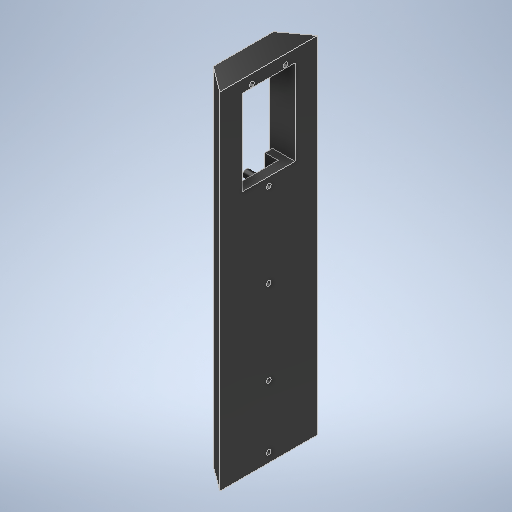
# Autodesk Inventor part: Fullenss sensor v3.1 holder
Saved by Autodesk Inventor 2025 (Build 290162000, 162)
## iProperties
Created: 2025-12-14
Part Number: Fullenss sensor v3.1 holder
Material: Generic
Document SubType Name: Modeling
Designer: kingc
Density: 1 g/cm^3
Appearance: Glossy - Black
Author: kingc
Autodesk Inventor part; units mm, degrees
ref_plane "YZ Plane" through (0, 0, 0) normal (1, 0, 0) x (0, 1, 0)
ref_plane "XZ Plane" through (0, 0, 0) normal (0, 1, 0) x (-1, 0, 0)
ref_plane "XY Plane" through (0, 0, 0) normal (0, 0, 1) x (1, 0, 0)
sketch "Sketch1" plane through (0, 0, 0) normal (1, 0, 0) x (0, 1, 0)
  line L0 (0, 0) -> (228.6, 0)
  line L1 (228.6, 0) -> (228.6, -35.56)
  line L2 (228.6, -35.56) -> (0, -35.56)
  line L3 (0, -35.56) -> (0, 0)
  line L4 (228.6, 0) -> (222.758, 0)
  line L5 (222.758, 0) -> (222.758, -35.56)
  line L6 (222.758, -35.56) -> (228.6, -35.56)
  line L7 (228.6, -35.56) -> (228.6, 0)
  circle A0 centre (224.79, -6.35) radius 1.5875
  circle A1 centre (224.79, -29.21) radius 1.5875
  line L8 (222.758, 0) -> (0, 0)
  line L9 (165.1, -5.08) -> (6.35, -5.08)
  line L10 (6.35, -5.08) -> (6.35, -30.48)
  line L11 (6.35, -30.48) -> (165.1, -30.48)
  line L12 (222.758, -33.02) -> (222.758, -2.54)
  line L13 (165.1, 0) -> (165.1, -35.56)
  line L14 (231.14, 2.54) -> (-2.54, 2.54)
  line L15 (-2.54, 2.54) -> (-2.54, -38.1)
  line L16 (-2.54, -38.1) -> (231.14, -38.1)
  line L17 (231.14, -38.1) -> (231.14, 2.54)
  point P0 (110.998, 0)
  point P1 (228.6, -17.78)
  dimension "d0" = 228.6
  dimension "d1" = 35.56
  dimension "d2" = 5.842
  dimension "d3" = 3.175
  dimension "d4" = 3.175
  dimension "d5" = 3.81
  dimension "d6" = 6.35
  dimension "d7" = 3.81
  dimension "d8" = 6.35
  dimension "d14" = 5.08
  dimension "d15" = 5.08
  dimension "d16" = 6.35
  dimension "d17" = 0
  dimension "d18" = 63.5
  dimension "d19" = 2.54
  dimension "d20" = 2.54
  dimension "d21" = 2.54
  dimension "d22" = 2.54
  constraints: 36 end point, 8 parallel, 7 point on line, 5 horizontal, 5 perpendicular, 2 centre point, 1 midpoint
  measures "d0" distance of L1.end L2.end
  measures "d1" distance of L0.end L1.end
  measures "d2" distance of L6.end L5.end
  measures "d3" diameter of A0
  measures "d4" diameter of A1
  measures "d5" distance from line of L1 A0.centre
  measures "d6" distance from line of L0 A0.centre
  measures "d7" distance from line of L1 A1.centre
  measures "d8" distance from line of L2 A1.centre
  measures "d14" distance between parallel lines of L0 L9
  measures "d15" distance between parallel lines of L2 L11
  measures "d16" distance between parallel lines of L3 L10
  measures "d17" distance between parallel lines of L5 L12
  measures "d18" distance from line of point (228.6, -17.78) L13
  measures "d19" distance between parallel lines of L14 L8
  measures "d20" distance between parallel lines of L16 L2
  measures "d21" distance between parallel lines of L15 L3
  measures "d22" distance between parallel lines of L17 L1
extrude "Extrusion1" add sketch "Sketch1" along normal blind 15.24 contours L0 L13 L9 L10 L11 L2 L3 | L0 L1 L2 L5
extrude "Extrusion2" add sketch "Sketch1" along normal blind 15.24 and the other way blind 2 contours L17 L16 L15 L14
sketch "Sketch2" plane through (15.24, 0, 0) normal (1, 0, 0) x (0, 0, -1)
  line L0 (5.08, 6.35) -> (5.08, 165.1) projected
  line L1 (30.48, 165.1) -> (30.48, 6.35) projected
  line L2 (30.48, 6.35) -> (5.08, 6.35) projected
  line L3 (5.08, 165.1) -> (30.48, 165.1)
  point P0 (0, 0)
  constraints: 2 end point, 1 horizontal
extrude "Extrusion3" add sketch "Sketch2" against normal blind 6.35
sketch "Sketch3" plane through (0, 0, 0) normal (-1, 0, 0) x (0, 0, 1)
  circle A0 centre (-17.78, 45.72) radius 2.54
  circle A1 centre (-17.78, 45.72) radius 1.5875
  line L0 (0, 228.6) -> (0, 0) projected
  line L1 (0, 0) -> (-35.56, 0) projected
  circle A2 centre (-17.78, 102.616) radius 2.54
  circle A3 centre (-17.78, 102.616) radius 1.5875
  circle A4 centre (-17.78, 159.512) radius 2.54
  circle A5 centre (-17.78, 159.512) radius 1.5875
  circle A6 centre (-17.78, 3.81) radius 1.5875
  dimension "d29" = 5.08
  dimension "d30" = 3.175
  dimension "d31" = 17.78
  dimension "d32" = 45.72
  dimension "d33" = 5.08
  dimension "d34" = 3.175
  dimension "d35" = 102.616
  dimension "d36" = 5.08
  dimension "d37" = 3.175
  dimension "d38" = 159.512
  dimension "d39" = 17.78
  dimension "d40" = 17.78
  dimension "d42" = 3.175
  constraints: 7 centre point, 3 coincident
  measures "d29" diameter of A0
  measures "d30" diameter of A1
  measures "d31" distance from line of L0 A0.centre
  measures "d32" distance from line of L1 A0.centre
  measures "d33" diameter of A2
  measures "d34" diameter of A3
  measures "d35" distance from line of L1 A2.centre
  measures "d36" diameter of A4
  measures "d37" diameter of A5
  measures "d38" distance from line of L1 A4.centre
  measures "d39" distance from line of L0 A4.centre
  measures "d40" distance from line of L0 A2.centre
  measures "d42" diameter of A6
extrude "Extrusion4" add sketch "Sketch3" against normal up to surface (8.89 mm away) contours A0 | A2 | A4
extrude "Extrusion5" cut sketch "Sketch3" against normal through all contours A1 | A3 | A5 | A6
sketch "Sketch4" plane through (-2, 231.14, 2.54) normal (0, 1, 0) x (1, 0, 0)
  line L0 (17.24, 40.64) -> (17.24, 0) projected
  line L1 (17.24, 0) -> (17.24, -12.7)
  line L2 (17.24, -12.7) -> (0, 0)
  line L3 (17.24, 40.64) -> (17.24, 53.34)
  line L4 (0, 40.64) -> (17.24, 40.64) projected
  line L5 (17.24, 53.34) -> (0, 40.64)
  line L6 (0, 0) -> (17.24, 0) projected
  point P0 (2, 2.54)
  dimension "d48" = 12.7
  dimension "d49" = 12.7
  constraints: 8 end point, 2 vertical
  measures "d48" distance of L0.end L1.end
  measures "d49" distance of L0.start L3.end
extrude "Extrusion6" add sketch "Sketch4" against normal up to surface (233.68 mm away)
body "Solid1"
